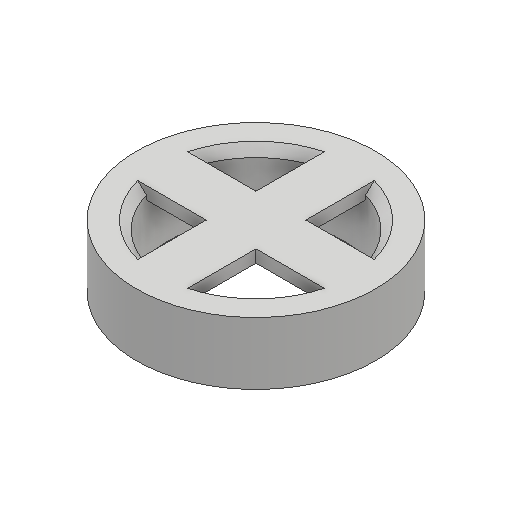
# Autodesk Inventor part: 3DP_PLA_Wheel_cover
Saved by Autodesk Inventor 2026.1 (Build 301233000, 233)
## iProperties
Created: 2016-05-27
Part Number: 3DP_PLA_Wheel_cover
Material: Ogólny
Document SubType Name: Modeling
Designer: Andrzej
Density: 1 g/cm^3
Appearance: Domyślna
Mass: 0.160641 g
Surface Area: 3.56595 cm^2
Volume: 0.160641 cm^3
Author: Andrzej
Autodesk Inventor part; units mm, degrees
ref_plane "YZ Plane" through (0, 0, 0) normal (1, 0, 0) x (0, 1, 0)
ref_plane "XZ Plane" through (0, 0, 0) normal (0, 1, 0) x (-1, 0, 0)
ref_plane "XY Plane" through (0, 0, 0) normal (0, 0, 1) x (1, 0, 0)
sketch "Szkic1" plane through (0, 0, 0) normal (0, 0, 1) x (1, 0, 0)
  circle A0 centre (0, 0) radius 5.75
  circle A1 centre (0, 0) radius 4.25
  dimension "d0" = 11.5
  dimension "d1" = 1.5
  constraints: 2 centre point, 1 coincident
  measures "d0" diameter of A0
  measures "d1" radial gap between concentric circles of A0 A1
extrude "Wyciągnięcie proste1" add sketch "Szkic1" along normal blind 0.6 contours A0 | A1
extrude "Wyciągnięcie proste2" add sketch "Szkic1" against normal blind 2.4
sketch "Szkic2" plane through (0, 0, 0.6) normal (0, 0, 1) x (1, 0, 0)
  circle A0 centre (0, 0) radius 5.75 projected
  circle A1 centre (0, 0) radius 4.25 projected
  line L0 (1.2, -4.0771) -> (1.2, -1.2)
  line L1 (1.2, 1.2) -> (1.2, 4.0771)
  line L2 (4.0771, -1.2) -> (1.2, -1.2)
  line L3 (-1.2, -1.2) -> (-4.0771, -1.2)
  line L4 (-1.2, -4.0771) -> (-1.2, -1.2)
  line L5 (-1.2, 1.2) -> (-1.2, 4.0771)
  line L6 (4.0771, 1.2) -> (1.2, 1.2)
  line L7 (-1.2, 1.2) -> (-4.0771, 1.2)
  constraints: 16 end point, 4 horizontal, 4 vertical, 9 other
extrude "Wyciągnięcie proste3" cut sketch "Szkic2" against normal through all contours L6 L1 A1 | A1 L0 L2 | L5 L7 A1 | A1 L3 L4
chamfer "Faza1" distance 0.4 angle 45 4 edges at (3.0052, -3.0052, 0.6) (3.0052, 3.0052, 0.6) (-3.0052, 3.0052, 0.6) (-3.0052, -3.0052, 0.6)
equation "\"d7\" = d6"
equation "\"d8\" = d6"
equation "\"d9\" = d6"
equation "\"d6\" = 1.2"
